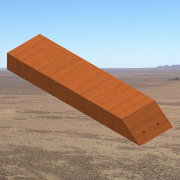
# Autodesk Inventor part: post_EdgeRimHoriz
Saved by Autodesk Inventor 2013 SP2 (Build 170200200, 200)
## iProperties
Created: 2013-09-06
Part Number: post_EdgeRimHoriz
Material: Wood (Cherry)
Document SubType Name: Modeling
Designer: Dave
Density: 0.5 g/cm^3
Mass: 635.373 g
Surface Area: 1042.45 cm^2
Volume: 1270.75 cm^3
Author: Dave
Autodesk Inventor part; units mm, degrees
ref_plane "YZ Plane" through (0, 0, 0) normal (1, 0, 0) x (0, 1, 0)
ref_plane "XZ Plane" through (0, 0, 0) normal (0, 1, 0) x (-1, 0, 0)
ref_plane "XY Plane" through (0, 0, 0) normal (0, 0, 1) x (1, 0, 0)
sketch "Sketch1" plane through (0, 0, 0) normal (0, 0, 1) x (1, 0, 0)
  line L0 (0, 0) -> (359.918, 0)
  line L1 (0, 0) -> (0, 38.1)
  line L2 (0, 38.1) -> (310.2651, 38.1)
  line L3 (359.918, 0) -> (310.2651, 38.1)
  dimension "d0" = 359.918
  dimension "d1" = 38.1
  dimension "d2" = 37.5
  constraints: 8 end point, 2 perpendicular
  measures "d0" distance of L0.start L0.end
  measures "d1" distance of L0.start L1.end
  measures "d2" angle of L3 L0
extrude "Extrusion1" add sketch "Sketch1" along normal blind 88.9
sketch "Sketch2" plane through (310.2651, 38.1, 88.9) normal (0.6087614, 0.7933533, 0) x (0.7933533, -0.6087614, 0)
  line L0 (62.5861, 88.9) -> (0, 88.9) projected
  line L1 (62.5861, 88.9) -> (62.5861, 0) projected
  circle A0 centre (43.5361, 63.5) radius 5.7238
  circle A1 centre (43.5361, 25.4) radius 5.7238
  point P0 (-222.9561, 88.9)
  dimension "d5" = 19.05
  dimension "d6" = 25.4
  dimension "d9" = 38.1
  constraints: 2 centre point, 1 vertical, 2 other
  measures "d5" distance from line of A0.centre L1
  measures "d6" distance from line of A0.centre L0
  measures "d9" distance of A0.centre A1.centre
hole "Hole1" at (344.8046, 11.5969, 63.5) at (344.8046, 11.5969, 25.4) direction (-0.6087614, -0.7933533, 0) diameter 6.35 end through all
body "Solid1"
